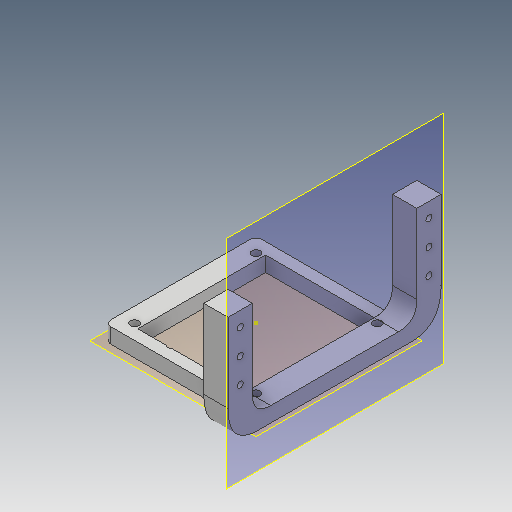
# Autodesk Inventor part: 30_Cube_LED_Array_v0
Saved by Autodesk Inventor 2019 (Build 230136000, 136)
## iProperties
Created: 2018-05-25
Part Number: 30_Cube_LED_Array_v0
Material: Generisch
Document SubType Name: Modeling
Designer: diederichbenedict
Density: 1 g/cm^3
Appearance: Vorgabe
Mass: 9.27173 g
Surface Area: 66.0193 cm^2
Volume: 9.27173 cm^3
Author: diederichbenedict
Autodesk Inventor part; units mm, degrees
ref_plane "YZ Plane" through (0, 0, 0) normal (1, 0, 0) x (0, 1, 0)
ref_plane "XZ Plane" through (0, 0, 0) normal (0, 1, 0) x (-1, 0, 0)
ref_plane "XY Plane" through (0, 0, 0) normal (0, 0, 1) x (1, 0, 0)
ref_plane "Arbeitsebene1" through (0, 0, 0) normal (0, 0, 1) x (1, 0, 0)
sketch "Skizze1" plane through (0, 0, 0) normal (0, 0, 1) x (1, 0, 0)
  arc A0 (13.4381, 5.6873) -> (13.3881, 5.2) centre (15.7881, 5.2) ccw construction
  line L0 (13.4381, 5.6873) -> (13.4381, 7.6) construction
  line L1 (13.4381, 7.6) -> (15.7881, 7.6) construction
  arc A1 (18.1881, 5.2) -> (15.7881, 7.6) centre (15.7881, 5.2) ccw projected
  line L2 (18.1881, 5.2) -> (18.1881, -5.2) construction
  arc A2 (15.7881, -7.6) -> (18.1881, -5.2) centre (15.7881, -5.2) ccw projected
  line L3 (15.7881, -7.6) -> (13.4381, -7.6) construction
  line L4 (13.4381, -7.6) -> (13.4381, -5.6873) construction
  arc A3 (13.3881, -5.2) -> (13.4381, -5.6873) centre (15.7881, -5.2) ccw construction
  line L5 (13.3881, -5.2) -> (13.3881, 5.2) construction
  arc A4 (14.5, 9) -> (11.5, 6) centre (14.5, 6) ccw construction
  line L6 (11.5, -6) -> (11.5, 6) construction
  arc A5 (11.5, -6) -> (14.5, -9) centre (14.5, -6) ccw construction
  line L7 (14.9, -9) -> (14.5, -9) construction
  arc A6 (17.9, -12) -> (14.9, -9) centre (14.9, -12) ccw projected
  line L8 (17.9, -12) -> (17.9, -21.066) projected
  line L9 (6.7383, -21.066) -> (-6.9383, -21.066) projected
  line L10 (-17.9, -21.066) -> (-17.9, 21.066) projected
  line L11 (-17.9, 21.066) -> (17.9, 21.066) projected
  line L12 (17.9, 21.066) -> (17.9, 12) projected
  arc A7 (14.9, 9) -> (17.9, 12) centre (14.9, 12) ccw projected
  line L13 (14.5, 9) -> (14.9, 9) construction
  circle A8 centre (-20, 20) radius 1.6 construction
  circle A9 centre (20, -20) radius 1.6 construction
  circle A10 centre (-20, -20) radius 1.6 construction
  circle A11 centre (20, 20) radius 1.6 construction
  arc A12 (-22.9, 24.9) -> (-24.9, 22.9) centre (-22.9, 22.9) ccw projected
  line L14 (-24.9, 22.9) -> (-24.9, -22.9) projected
  arc A13 (-24.9, -22.9) -> (-22.9, -24.9) centre (-22.9, -22.9) ccw projected
  line L15 (-22.9, -24.9) -> (22.9, -24.9) projected
  arc A14 (22.9, -24.9) -> (24.9, -22.9) centre (22.9, -22.9) ccw projected
  line L16 (24.9, -22.9) -> (24.9, 22.9) projected
  arc A15 (24.9, 22.9) -> (22.9, 24.9) centre (22.9, 22.9) ccw projected
  line L17 (22.9, 24.9) -> (-22.9, 24.9) projected
  arc A16 (6.7383, -21.066) -> (8.3017, -21.066) centre (7.52, -20.62) ccw projected
  arc A17 (-8.5017, -21.066) -> (-6.9383, -21.066) centre (-7.72, -20.62) ccw projected
  line L18 (-8.5017, -21.066) -> (-17.9, -21.066) projected
  line L19 (17.9, -21.066) -> (8.3017, -21.066) projected
  line L20 (17.9, -12) -> (17.9, 12)
  circle A18 centre (-20, 20) radius 1.4
  line L21 (-20, 20) -> (20, 20) construction
  line L22 (20, 20) -> (20, -20) construction
  line L23 (20, -20) -> (-20, -20) construction
  line L24 (-20, -20) -> (-20, 20) construction
  circle A19 centre (20, -20) radius 1.4
  circle A20 centre (20, 20) radius 1.4
  circle A21 centre (-20, -20) radius 1.4
  line L25 (25.9, -32.5) -> (25.9, 32.5) projected
  line L26 (22.9, -24.9) -> (25.9, -24.9)
  line L27 (22.9, 24.9) -> (25.9, 24.9)
  point P0 (0, 0)
  dimension "d7" = 2.8
  dimension "d8" = 40
  dimension "d9" = 40
  dimension "d10" = 2.8
  dimension "d11" = 2.8
  dimension "d12" = 2.8
  constraints: 14 end point, 4 centre point, 4 coincident, 3 perpendicular, 2 parallel, 2 point on line, 1 horizontal, 1 point on circle, 1 vertical
  measures "d7" diameter of A18
  measures "d8" distance of L22.end L23.end
  measures "d9" distance of L21.end L22.end
  measures "d10" diameter of A19
  measures "d11" diameter of A20
  measures "d12" diameter of A21
extrude "Extrusion1" add sketch "Skizze1" along normal blind 5
sketch "Skizze2" plane through (0, 0, 5) normal (0, 0, 1) x (1, 0, 0)
  point P0 (0, 0)
ref_plane "Arbeitsebene2" through (25.9, 0, 24.2) normal (-1, 0, 0) x (0, 0, 1)
sketch "Skizze3" plane through (25.9, 0, 24.2) normal (-1, 0, 0) x (0, 0, 1)
  circle A0 centre (-31.1, -8.2) radius 1 projected
  circle A1 centre (31.1, 8.2) radius 1 projected
  circle A2 centre (-31.1, 0) radius 1 projected
  circle A3 centre (31.1, 0) radius 1 projected
  circle A4 centre (31.1, -8.2) radius 1 projected
  circle A5 centre (-31.1, 8.2) radius 1 projected
  circle A6 centre (8.2, 31.1) radius 1 projected
  circle A7 centre (-8.2, -31.1) radius 1 projected
  circle A8 centre (0, -31.1) radius 1 projected
  circle A9 centre (0, 31.1) radius 1 projected
  circle A10 centre (8.2, -31.1) radius 1 projected
  circle A11 centre (-8.2, 31.1) radius 1 projected
  circle A12 centre (0, 0) radius 0.75 projected
  line L0 (-32.5, 32.5) -> (32.5, 32.5) projected
  line L1 (-32.5, -32.5) -> (-32.5, 32.5) projected
  line L2 (32.5, -32.5) -> (-32.5, -32.5) projected
  line L3 (32.5, 32.5) -> (32.5, -32.5) projected
  line L4 (-19.2, 22.9) -> (-19.2, -22.9) construction
  line L5 (-19.2, 0) -> (31.1, 0) construction
  line L6 (-13, -35.1) -> (13, -35.1)
  line L7 (13, -35.1) -> (13, -27.1)
  line L8 (13, -27.1) -> (-13, -27.1)
  line L9 (-13, -27.1) -> (-13, -35.1)
  line L10 (-13, -35.1) -> (13, -27.1) construction
  line L11 (13, -35.1) -> (-13, -27.1) construction
  line L12 (-24.2, -21.066) -> (-19.2, -21.066) projected
  line L13 (-24.2, -24.9) -> (-19.2, -24.9) projected
  line L14 (-19.2, -22.9) -> (-19.2, 22.9) projected
  line L15 (-19.2, 21.066) -> (-19.2, -21.066) projected
  line L16 (-19.2, 0) -> (-19.2, -21.066)
  line L17 (-24.2, -22.9) -> (-19.2, -22.9) projected
  line L18 (-19.2, -21.066) -> (-19.2, -22.9)
  line L19 (-19.2, -22.9) -> (-24.2, -22.9)
  line L20 (-24.2, 22.9) -> (-24.2, -22.9) projected
  line L21 (-24.2, -24.9) -> (-19.2, -24.9) projected
  line L22 (-24.2, -22.9) -> (-24.2, -24.9)
  line L23 (-19.2, -24.9) -> (-19.2, -22.9) projected
  line L24 (-24.2, -24.9) -> (-24.2, -35.1) construction
  line L25 (-24.2, -35.1) -> (-13, -35.1) construction
  spline S0 degree 2 poles (-24.2, -24.9) (-24.2, -35.1) (-13, -35.1) knots 1 1 1 2 2 2
  line L26 (-19.2, -21.066) -> (-19.2, -27.1) construction
  line L27 (-19.2, -27.1) -> (-13, -27.1) construction
  spline S1 degree 2 poles (-19.2, -21.066) (-19.2, -27.1) (-13, -27.1) knots 1 1 1 2 2 2
  circle A13 centre (-8.2, 31.1) radius 1
  circle A14 centre (0, 31.1) radius 1
  circle A15 centre (8.2, 31.1) radius 1
  line L28 (-13, 35.1) -> (13, 35.1)
  line L29 (13, 35.1) -> (13, 27.1)
  line L30 (13, 27.1) -> (-13, 27.1)
  line L31 (-13, 27.1) -> (-13, 35.1)
  line L32 (-13, 35.1) -> (13, 27.1) construction
  line L33 (13, 35.1) -> (-13, 27.1) construction
  line L34 (-24.2, 21.066) -> (-19.2, 21.066)
  line L35 (-24.2, 24.9) -> (-19.2, 24.9)
  line L36 (-24.2, 22.9) -> (-19.2, 22.9)
  line L37 (-19.2, 21.066) -> (-19.2, 22.9)
  line L38 (-19.2, 22.9) -> (-24.2, 22.9)
  line L39 (-24.2, 24.9) -> (-19.2, 24.9)
  line L40 (-24.2, 22.9) -> (-24.2, 24.9)
  line L41 (-19.2, 24.9) -> (-19.2, 22.9)
  line L42 (-24.2, 24.9) -> (-24.2, 35.1) construction
  line L43 (-24.2, 35.1) -> (-13, 35.1) construction
  spline S2 degree 2 poles (-24.2, 24.9) (-24.2, 35.1) (-13, 35.1) knots 1 1 1 2 2 2
  line L44 (-19.2, 21.066) -> (-19.2, 27.1) construction
  line L45 (-19.2, 27.1) -> (-13, 27.1) construction
  spline S3 degree 2 poles (-19.2, 21.066) (-19.2, 27.1) (-13, 27.1) knots 1 1 1 2 2 2
  point P0 (-24.2, 0)
  dimension "d2" = 26
  dimension "d3" = 8
  constraints: 50 end point, 12 symmetric about line, 6 midpoint, 4 perpendicular, 3 parallel, 2 collinear, 15 other
  measures "d2" distance of L6.start L6.end
  measures "d3" distance of L7.end L6.end
extrude "Extrusion2" add sketch "Skizze3" along normal up to surface (8 mm away) contours S2 L31 L0 | L0 L31 S3 L14 L41 L35 S2 | L31 L28 L29 L0 | L0 L29 L30 L31 | S0 L13 L23 L14 S1 L9 L2 | L2 L9 S0 | L9 L8 L7 L2 | L2 L7 L6 L9 | L22 L17 L23 L13
